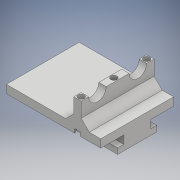
# Autodesk Inventor part: CarroXY - Hotend
Saved by Autodesk Inventor 2017 (Build 210142000, 142)
## iProperties
Created: 2020-08-23
Part Number: CarroXY - Hotend
Material: Generic
Document SubType Name: Modeling
Designer: ale
Density: 1 g/cm^3
Appearance: Default
Author: ale
Autodesk Inventor part; units mm, degrees
ref_plane "YZ Plane" through (0, 0, 0) normal (1, 0, 0) x (0, 1, 0)
ref_plane "XZ Plane" through (0, 0, 0) normal (0, 1, 0) x (-1, 0, 0)
ref_plane "XY Plane" through (0, 0, 0) normal (0, 0, 1) x (1, 0, 0)
sketch "Sketch2" plane through (0, 0, 0) normal (1, 0, 0) x (0, 1, 0)
  line L0 (-19.9252, 0) -> (19.9252, 0)
  line L1 (0, -28.9507) -> (0, 28.9507)
  line L2 (14.5, -7.3) -> (-14.5, -7.3)
  line L3 (-14.5, -7.3) -> (-14.5, -3)
  line L4 (-10, -3) -> (-10, 3)
  line L5 (-27, 3) -> (-27, 9)
  line L6 (-27, 9) -> (27, 9)
  line L7 (14.5, -7.3) -> (14.5, -3)
  line L8 (10, -3) -> (10, 3)
  line L9 (27, 3) -> (27, 9)
  line L10 (-14.5, -3) -> (-10, -3)
  line L11 (10, -3) -> (14.5, -3)
  line L12 (27, 3) -> (10, 3)
  line L13 (-10, 3) -> (-27, 3)
  point P0 (0, 0)
  point P1 (0, 0)
  point P2 (10, 0)
  dimension "d4" = 14.5
  dimension "d8" = 27
  dimension "d9" = 10
  dimension "d10" = 4.3
  dimension "d11" = 6
  dimension "d12" = 6
  constraints: 28 end point, 10 perpendicular, 6 symmetric about line, 3 midpoint, 2 horizontal, 1 coincident, 1 point on line, 1 vertical
  measures "d4" distance between parallel lines of L3 L1
  measures "d8" distance between parallel lines of L5 L1
  measures "d9" distance between parallel lines of L4 L1
  measures "d10" distance between parallel lines of L10 L2
  measures "d11" distance between parallel lines of L13 L10
  measures "d12" distance between parallel lines of L6 L13
extrude "Extrusion2" add sketch "Sketch2" along normal blind 70
sketch "Sketch3" plane through (0, -27, 9) normal (0, 0, 1) x (1, 0, 0)
  line L0 (0, 0) -> (70, 0) projected
  line L1 (0, 54) -> (70, 54) projected
  line L2 (55.5, 0) -> (50, 0)
  line L3 (50, 0) -> (50, 54)
  line L4 (50, 54) -> (55.5, 54)
  line L5 (55.5, 54) -> (55.5, 0)
  line L6 (70, 54) -> (70, 0) projected
  point P0 (0, 27)
  dimension "d15" = 20
  dimension "d16" = 5.5
  constraints: 8 end point, 2 parallel, 2 point on line, 1 horizontal, 1 perpendicular
  measures "d15" distance between parallel lines of L6 L3
  measures "d16" distance between parallel lines of L3 L5
extrude "Extrusion3" add sketch "Sketch3" along normal blind 17 contours L3 L1 L5 L0
sketch "Sketch4" plane through (50, -27, 9) normal (-1, 0, 0) x (0, 0, 1)
  line L0 (17, 54) -> (17, 0) projected
  circle A0 centre (17, 42) radius 6.5
  circle A1 centre (17, 12) radius 6.5
  line L1 (0, 0) -> (17, 0) projected
  point P0 (-9, 27)
  dimension "d19" = 13
  dimension "d20" = 13
  dimension "d21" = 30
  dimension "d22" = 12
  constraints: 2 centre point, 2 point on line
  measures "d19" diameter of A0
  measures "d20" diameter of A1
  measures "d21" distance of A0.centre A1.centre
  measures "d22" distance from line of L1 A1.centre
extrude "Extrusion4" cut sketch "Sketch4" against normal up to surface (5.5 mm away)
sketch "Sketch5" plane through (0, -14.5, -7.3) normal (0, 0, -1) x (-1, 0, 0)
  line L0 (0, 0) -> (-70, 0)
  line L1 (-55.5, 29) -> (-55.5, 0)
  line L2 (-50, 0) -> (-50, 29)
  line L3 (-50, 14.5) -> (-55.5, 14.5)
  line L4 (-50, -12.5) -> (-50, 41.5) projected
  line L5 (-55.5, 41.5) -> (-55.5, -12.5) projected
  line L6 (0, -12.5) -> (-70, -12.5) projected
  point P0 (0, 27)
  point P1 (-52.75, -9.75)
  point P2 (-52.75, 14.5)
  point P3 (-52.75, 38.75)
  dimension "d26" = 2.75
  dimension "d34" = 2.75
  constraints: 8 end point, 5 midpoint, 1 symmetric about line
  measures "d26" distance from line of L1 point (-52.75, -9.75)
  measures "d34" distance from line of L6 point (-52.75, -9.75)
hole "Hole1" at (52.75, -24.25, -7.3) at (52.75, 0, -7.3) at (52.75, 24.25, -7.3) direction (0, 0, 1) diameter 4.5 end through all
sketch "Sketch6" plane through (0, -14.5, -7.3) normal (0, 0, -1) x (-1, 0, 0)
  circle A0 centre (-52.75, 14.5) radius 2.25 projected
  line L0 (-56.25, 14.5) -> (-54.5, 17.5311)
  line L1 (-54.5, 17.5311) -> (-51, 17.5311)
  line L2 (-51, 17.5311) -> (-49.25, 14.5)
  line L3 (-49.25, 14.5) -> (-51, 11.4689)
  line L4 (-51, 11.4689) -> (-54.5, 11.4689)
  line L5 (-54.5, 11.4689) -> (-56.25, 14.5)
  circle A1 centre (-52.75, 38.75) radius 2.25 projected
  line L6 (-56.25, 38.75) -> (-54.5, 41.7811)
  line L7 (-54.5, 41.7811) -> (-51, 41.7811)
  line L8 (-51, 41.7811) -> (-49.25, 38.75)
  line L9 (-49.25, 38.75) -> (-51, 35.7189)
  line L10 (-51, 35.7189) -> (-54.5, 35.7189)
  line L11 (-54.5, 35.7189) -> (-56.25, 38.75)
  circle A2 centre (-52.75, -9.75) radius 2.25 projected
  line L12 (-56.25, -9.75) -> (-54.5, -6.7189)
  line L13 (-54.5, -6.7189) -> (-51, -6.7189)
  line L14 (-51, -6.7189) -> (-49.25, -9.75)
  line L15 (-49.25, -9.75) -> (-51, -12.7811)
  line L16 (-51, -12.7811) -> (-54.5, -12.7811)
  line L17 (-54.5, -12.7811) -> (-56.25, -9.75)
  point P0 (0, 14.5)
  dimension "d35" = 7
  dimension "d36" = 7
  dimension "d37" = 7
  constraints: 36 end point, 3 coincident, 39 other
  measures "d35" distance of L0.start L2.end
  measures "d36" distance of L6.start L8.end
  measures "d37" distance of L12.start L14.end
extrude "Extrusion5" cut sketch "Sketch6" against normal blind 13.3
chamfer "Chamfer1" distance 6 angle 45 2 edges at (50, 0, 9) (55.5, 0, 9)
equation "\"d23\" = d21"
body "Solid2"
